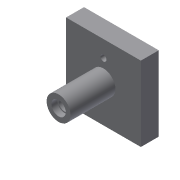
# Autodesk Inventor part: Base
Saved by Autodesk Inventor 2017 (Build 210142000, 142)
## iProperties
Created: 2016-07-28
Part Number: Base
Material: Generic
Document SubType Name: Modeling
Designer: Tutorial Books
Density: 1 g/cm^3
Appearance: Default
Author: Tutorial Books
Autodesk Inventor part; units mm, degrees
ref_plane "YZ Plane" through (0, 0, 0) normal (1, 0, 0) x (0, 1, 0)
ref_plane "XZ Plane" through (0, 0, 0) normal (0, 1, 0) x (-1, 0, 0)
ref_plane "XY Plane" through (0, 0, 0) normal (0, 0, 1) x (1, 0, 0)
ref_plane "Work Plane1" through (0, 0, 0) normal (0, 0, 1) x (1, 0, 0)
sketch "Sketch1" plane through (0, 0, 0) normal (0, 0, 1) x (1, 0, 0)
  line L0 (79.375, 79.375) -> (-79.375, 79.375)
  line L1 (-79.375, 79.375) -> (-79.375, -79.375)
  line L2 (-79.375, -79.375) -> (79.375, -79.375)
  line L3 (79.375, -79.375) -> (79.375, 79.375)
  line L4 (79.375, 79.375) -> (-79.375, -79.375) construction
  line L5 (-79.375, 79.375) -> (79.375, -79.375) construction
  point P0 (0, 0)
  dimension "d0" = 158.75
  dimension "d1" = 158.75
  constraints: 12 end point, 2 midpoint, 2 parallel, 1 horizontal, 1 perpendicular
  measures "d0" distance of L1.end L2.end
  measures "d1" distance of L0.end L1.end
extrude "Extrusion1" add sketch "Sketch1" along normal blind 38.1
sketch "Sketch2" plane through (0, 0, 38.1) normal (0, 0, 1) x (1, 0, 0)
  circle A0 centre (0, 0) radius 25.4
  dimension "d4" = 50.8
  constraints: 1 centre point, 1 coincident
  measures "d4" diameter of A0
extrude "Extrusion2" add sketch "Sketch2" along normal blind 95.25
hole "Hole1" at (0, 0, 133.35) direction (0, 0, -1) diameter 25.4 end through all counterbore diameter 30.48 counterbore depth 12.7
sketch "Sketch3" plane through (0, 0, 38.1) normal (0, 0, 1) x (1, 0, 0)
  circle A0 centre (0, 0) radius 12.7 construction
  circle A1 centre (0, 0) radius 44.45 construction
  point P0 (0, 44.45)
  dimension "d16" = 88.9
  constraints: 1 coincident, 1 vertical alignment, 2 other
hole "Hole2" at (0, 44.45, 38.1) direction (0, 0, -1) diameter 12.7 end through all
pattern_circular "Circular Pattern1" count 4 over 360 about axis through (0, 0, 38.1) along (0, 0, 1) of "Hole2"
body "Solid1"
